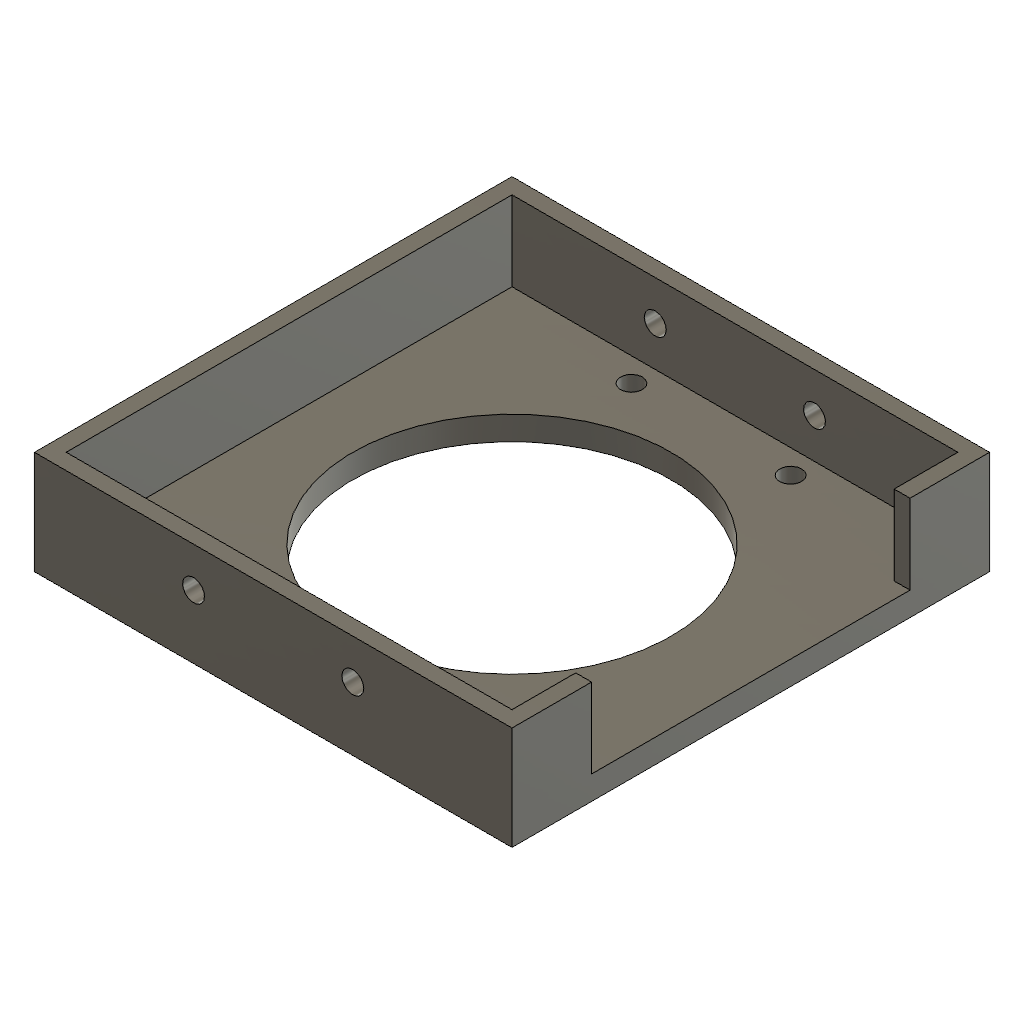
TankBot Lidar Base (Autodesk Fusion 360 design; units mm, degrees)
Autodesk Fusion 360 part; units mm, degrees
box "BoxPrimitive1" add length 60 width 60 height 20 placed x (0, 0, 1) y (1, 0, 0) z (0, 1, 0) at (0, 0, -1.7806)
shell "Shell1" thickness 2 removed faces 1 at (40, 20, 18.2194)
box "BoxPrimitive2" add length 35 width 2 height 1 placed x (0, 0, -1) y (-1, 0, 0) z (0, 1, 0) at (60, 20, 50)
extrude "Extrude1" add 1 faces at (59.3333, 20.3333, 15) along direction (0, 0, -1) blind 6.781
extrude "Extrude2" cut 1 faces at (59.3333, 20.3333, 50) along direction (0, 0, -1) blind 1.781
extrude "Extrude3" cut 1 faces at (58.6667, 21, 21.5523) along direction (0, -1, 0) blind 19
extrude "Extrude4" cut 1 faces at (0.6667, 20, 37.5527) along direction (0, -1, 0) blind 8
hole "Hole1" at (40, 0, 53.2194) direction (0, 1, 0) diameter 2.75 depth 3 tip angle 180
hole "Hole2" at (20, 0, 53.2194) direction (0, 1, 0) diameter 2.75 depth 3 tip angle 180
hole "Hole3" at (40, 0, 3.2194) direction (0, 1, 0) diameter 2.75 depth 3 tip angle 180
hole "Hole4" at (20, 0, 3.2194) direction (0, 1, 0) diameter 2.75 depth 3 tip angle 180
extrude "Extrude5" add 1 faces at (53.5915, 0, 36.174) along direction (0, -1, 0) blind 1
hole "Hole5" at (20, 7, 58.2194) direction (0, 0, -1) diameter 2.75 depth 3 tip angle 180
hole "Hole6" at (40, 7, 58.2194) direction (0, 0, -1) diameter 2.75 depth 3 tip angle 180
hole "Hole7" at (20, 7, -1.7806) direction (0, 0, 1) diameter 2.75 depth 3 tip angle 180
hole "Hole8" at (40, 7, -1.7806) direction (0, 0, 1) diameter 2.75 depth 3 tip angle 180
hole "Hole9" at (30, 2, 28.2194) direction (0, -1, 0) diameter 40 depth 3 tip angle 180
